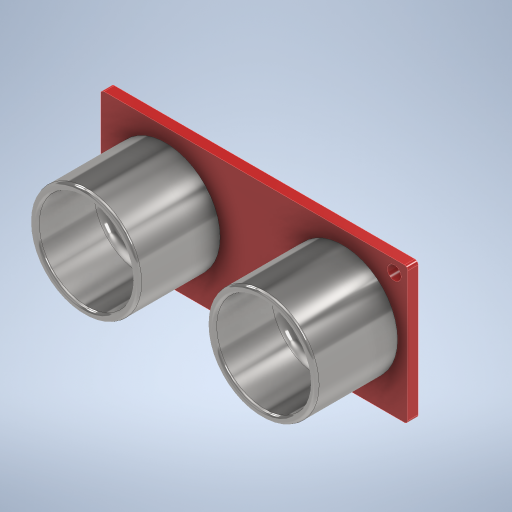
# Autodesk Inventor part: US
Saved by Autodesk Inventor 2023 (Build 270158000, 158)
## iProperties
Created: 2022-07-24
Part Number: US
Material: Genérico
Document SubType Name: Modeling
Designer: LJNC
Density: 1 g/cm^3
Appearance: Valor por defecto
Author: LJNC
Autodesk Inventor part; units mm, degrees
ref_plane "YZ Plane" through (0, 0, 0) normal (1, 0, 0) x (0, 1, 0)
ref_plane "XZ Plane" through (0, 0, 0) normal (0, 1, 0) x (-1, 0, 0)
ref_plane "XY Plane" through (0, 0, 0) normal (0, 0, 1) x (1, 0, 0)
sketch "Boceto1" plane through (0, 0, 0) normal (0, 0, 1) x (1, 0, 0)
  line L0 (-22.5, 10) -> (22.5, 10)
  line L1 (22.5, 10) -> (22.5, -10)
  line L2 (22.5, -10) -> (-22.5, -10)
  line L3 (-22.5, -10) -> (-22.5, 10)
  line L4 (-22.5, 0) -> (22.5, 0) construction
  circle A0 centre (-13, 0) radius 8
  circle A1 centre (13, 0) radius 8
  circle A2 centre (-20.5, -8.25) radius 1
  circle A3 centre (20.5, 8.25) radius 1
  circle A4 centre (-13, 0) radius 7
  circle A5 centre (13, 0) radius 7
  point P0 (0, 0)
  point P1 (0, 0)
  dimension "d0" = 45
  dimension "d1" = 20
  dimension "d2" = 16
  dimension "d3" = 13
  dimension "d4" = 13
  dimension "d5" = 2
  dimension "d6" = 20.5
  dimension "d7" = 8.25
  dimension "d8" = 8.25
  dimension "d9" = 20.5
  dimension "d14" = 1
  constraints: 10 end point, 6 centre point, 3 coincident, 3 equal radius, 3 midpoint, 2 parallel, 2 point on line, 1 horizontal, 1 perpendicular
  measures "d0" distance of L0.start L0.end
  measures "d1" distance of L0.end L1.end
  measures "d2" diameter of A0
  measures "d3" distance of point (0, 0) A0.centre
  measures "d4" distance of point (0, 0) A1.centre
  measures "d5" diameter of A2
  measures "d6" horizontal distance of point (0, 0) A2.centre
  measures "d7" vertical distance of A0.centre A2.centre
  measures "d8" distance from line of L4 A3.centre
  measures "d9" horizontal distance of point (0, 0) A3.centre
  measures "d14" radial gap between concentric circles of A0 A4
extrude "Extrusión1" add sketch "Boceto1" along normal blind 12 contours A0 | A1
extrude "Extrusión2" add sketch "Boceto1" against normal blind 1.5 separate body contours L0 L1 L2 L3 | A0 | A1 | A4 | A5
fillet "Empalme2" radius 0.5 4 edges at (-21, 0, 12) (-20, 0, 12) (5, 0, 12) (6, 0, 12)
extrude "Extrusión3" add sketch "Boceto1" along normal blind 1.5 contours A4 | A5 bodies 1
fillet "Empalme3" radius 2 2 edges at (-20, 0, 1.5) (6, 0, 1.5)
fillet "Empalme4" radius 0.5 4 edges at (-22.5, 10, -0.75) (-22.5, -10, -0.75) (22.5, -10, -0.75) (22.5, 10, -0.75)
sketch "Boceto2" plane through (0, 0, -1.5) normal (0, 0, -1) x (-1, 0, 0)
  line L0 (-5.25, -7) -> (5.25, -7)
  line L1 (5.25, -7) -> (5.25, -9.5)
  line L2 (5.25, -9.5) -> (-5.25, -9.5)
  line L3 (-5.25, -9.5) -> (-5.25, -7)
  line L4 (0, 0) -> (0, -7) construction
  arc A0 (-22, 10) -> (-22.5, 9.5) centre (-22, 9.5) ccw construction
  line L5 (-22.5, 9.5) -> (-22.5, -9.5) construction
  arc A1 (-22.5, -9.5) -> (-22, -10) centre (-22, -9.5) ccw construction
  line L6 (-22, -10) -> (22, -10) construction
  arc A2 (22, -10) -> (22.5, -9.5) centre (22, -9.5) ccw construction
  line L7 (22.5, -9.5) -> (22.5, 9.5) construction
  arc A3 (22.5, 9.5) -> (22, 10) centre (22, 9.5) ccw construction
  line L8 (22, 10) -> (-22, 10) construction
  circle A4 centre (-20.5, 8.25) radius 1 construction
  circle A5 centre (20.5, -8.25) radius 1 construction
  dimension "d21" = 10.5
  dimension "d22" = 2.5
  dimension "d23" = 0.5
  constraints: 10 end point, 2 parallel, 1 horizontal, 1 midpoint, 1 perpendicular, 1 vertical
  measures "d21" distance of L0.start L0.end
  measures "d22" distance of L0.end L1.end
  measures "d23" distance between parallel lines of L6 L2
extrude "Extrusión4" add sketch "Boceto2" along normal blind 2.5 separate body
sketch "Boceto3" plane through (0, 0, -4) normal (0, 0, -1) x (-1, 0, 0)
  line L0 (-5.25, -9.5) -> (5.25, -9.5) construction
  line L1 (5.25, -9.5) -> (5.25, -7) construction
  line L2 (5.25, -7) -> (-5.25, -7) construction
  line L3 (-5.25, -7) -> (-5.25, -9.5) construction
  line L4 (-4.2375, -7.95) -> (-3.6375, -7.95)
  line L5 (-3.6375, -7.95) -> (-3.6375, -8.55)
  line L6 (-3.6375, -8.55) -> (-4.2375, -8.55)
  line L7 (-4.2375, -8.55) -> (-4.2375, -7.95)
  line L8 (-5.25, -8.25) -> (5.25, -8.25) construction
  line L9 (-3.9375, -8.55) -> (-3.9375, -7.95) construction
  line L10 (-1.6125, -7.95) -> (-1.0125, -7.95)
  line L11 (-1.0125, -7.95) -> (-1.0125, -8.55)
  line L12 (-1.0125, -8.55) -> (-1.6125, -8.55)
  line L13 (-1.6125, -8.55) -> (-1.6125, -7.95)
  line L14 (-1.3125, -8.55) -> (-1.3125, -7.95) construction
  point P0 (0, 0)
  point P1 (-4.2375, -8.25)
  point P2 (-1.6125, -8.25)
  dimension "d26" = 0.6
  dimension "d27" = 10.5
  dimension "d28" = 1.3125
  dimension "d30" = 2.625
  constraints: 22 end point, 8 midpoint, 4 parallel, 3 equal length, 2 horizontal, 2 perpendicular, 2 point on line
  measures "d26" distance of L4.start L4.end
  measures "d27" distance of L1.end L2.end
  measures "d28" distance between parallel lines of L3 L9
  measures "d30" distance between parallel lines of L9 L14
extrude "Extrusión5" add sketch "Boceto3" along normal blind 8.5 separate body
fillet "Empalme5" radius 0.1 16 edges at (4.2375, -7.95, -8.25) (3.6375, -7.95, -8.25) (3.6375, -8.55, -8.25) (4.2375, -8.55, -8.25) (4.2375, -8.25, -12.5) (3.6375, -8.25, -12.5) (3.9375, -7.95, -12.5) (3.9375, -8.55, -12.5) (1.6125, -7.95, -8.25) (1.6125, -8.55, -8.25) (1.0125, -7.95, -8.25) (1.0125, -8.55, -8.25) (1.0125, -8.25, -12.5) (1.3125, -7.95, -12.5) (1.6125, -8.25, -12.5) (1.3125, -8.55, -12.5)
fillet "Empalme6" radius 0.5 8 edges at (0, -7, -4) (0, -9.5, -4) (-5.25, -8.25, -4) (-5.25, -7, -2.75) (-5.25, -9.5, -2.75) (5.25, -9.5, -2.75) (5.25, -7, -2.75) (5.25, -8.25, -4)
mirror "Simetría1" about plane through (0, 0, 0) normal (1, 0, 0) bodies 4
equation "\"d4\" = d3"
equation "\"d8\" = d7"
equation "\"d9\" = d6"
equation "\"d28\" = 0.125 * d27"
equation "\"d30\" = 2 * d28"
